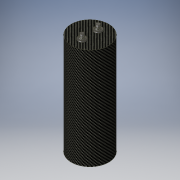
# Autodesk Inventor part: 3.5F_Cap
Saved by Autodesk Inventor 2016 (Build 200138000, 138)
## iProperties
Created: 2016-05-08
Part Number: 3.5F_Cap
Material: Aluminum 6061
Document SubType Name: Modeling
Designer: agmle
Density: 2.7 g/cm^3
Appearance: Carbon Fiber 1
Mass: 5728.15 g
Surface Area: 1015.64 cm^2
Volume: 2121.54 cm^3
Diameter: 3.934 in
Length: 10.630 in
Author: agmle
Autodesk Inventor part; units mm, degrees
ref_plane "YZ Plane" through (0, 0, 0) normal (1, 0, 0) x (0, 1, 0)
ref_plane "XZ Plane" through (0, 0, 0) normal (0, 1, 0) x (-1, 0, 0)
ref_plane "XY Plane" through (0, 0, 0) normal (0, 0, 1) x (1, 0, 0)
sketch "Sketch1" plane through (0, 0, 0) normal (0, 1, 0) x (-1, 0, 0)
  circle A0 centre (0, 0) radius 49.9618
  dimension "Diameter" = 99.9236
  constraints: 1 centre point, 1 coincident
  measures "Diameter" diameter of A0
extrude "Extrusion1" add sketch "Sketch1" along normal blind 270
sketch "Sketch2" plane through (0, 270, 0) normal (0, 1, 0) x (1, 0, 0)
  circle A0 centre (0, -21.3551) radius 9.9758
  circle A1 centre (0, 21.3551) radius 9.9758
  line L0 (0, -21.3551) -> (0, 21.3551) construction
  point P0 (0, 0)
  point P1 (0, 0)
  dimension "d3" = 19.9517
  dimension "d6" = 42.7101
  constraints: 2 centre point, 2 end point, 1 coincident, 1 equal radius, 1 midpoint, 1 vertical
  measures "d3" diameter of A0
  measures "d6" distance of L0.start L0.end
extrude "Extrusion2" add sketch "Sketch2" along normal blind 3.3528
sketch "Sketch3" plane through (0, 273.3528, 21.3551) normal (0, 1, 0) x (1, 0, 0)
  circle A0 centre (0, 42.7101) radius 9.9758 construction
  circle A1 centre (0, 0) radius 9.9758 construction
  circle A2 centre (0, 42.7101) radius 6.731
  circle A3 centre (0, 0) radius 6.731
  point P0 (0, 21.3551)
  dimension "d7" = 13.462
  constraints: 2 centre point, 2 coincident, 1 equal radius
  measures "d7" diameter of A2
extrude "Extrusion3" add sketch "Sketch3" along normal blind 3.175
sketch "Sketch4" plane through (0, 276.5278, 21.3551) normal (0, 1, 0) x (1, 0, 0)
  circle A0 centre (0, 42.7101) radius 6.731 construction
  circle A1 centre (0, 0) radius 6.731 construction
  circle A2 centre (0, 42.7101) radius 5.4229
  circle A3 centre (0, 0) radius 5.4229
  point P0 (0, 21.3551)
  dimension "d10" = 10.8458
  constraints: 2 centre point, 2 coincident, 1 equal radius
  measures "d10" diameter of A2
extrude "Extrusion4" add sketch "Sketch4" along normal blind 2.794
sketch "Sketch5" plane through (0, 279.3218, 21.3551) normal (0, 1, 0) x (1, 0, 0)
  circle A0 centre (0, 42.7101) radius 5.4229 construction
  circle A1 centre (0, 0) radius 5.4229 construction
  circle A2 centre (0, 42.7101) radius 4.6164
  circle A3 centre (0, 0) radius 4.6164
  point P0 (0, 21.3551)
  dimension "d13" = 9.2329
  constraints: 2 centre point, 2 coincident, 1 equal radius
  measures "d13" diameter of A2
extrude "Extrusion5" add sketch "Sketch5" along normal blind 5.4864
thread "Thread1" size "9/16-28 UN" class "2A" standard "ANSI Unified Screw Threads" full length
thread "Thread2" size "9/16-28 UN" class "2A" standard "ANSI Unified Screw Threads" full length
chamfer "Chamfer1" distance 0.9525 angle 45 2 edges at (-6.731, 276.5278, -21.3551) (-6.731, 276.5278, 21.3551)
chamfer "Chamfer2" distance 0.6223 angle 45 2 edges at (-5.4229, 279.3218, 21.3551) (-5.4229, 279.3218, -21.3551)
body "Solid1"
